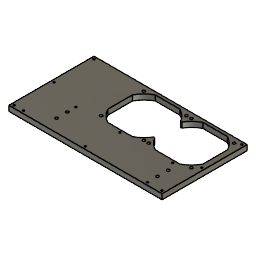
back (Autodesk Fusion 360 design; units mm, degrees)
Autodesk Fusion 360 part; units mm, degrees
sketch "Skizze1" plane through (0, 0, 0) normal (0, 0, 1) x (1, 0, 0)
  line L0 (258, 143.5) -> (0, 143.5)
  circle A0 centre (229, 39.5) radius 2.25
  circle A1 centre (229, 21.5) radius 2.25
  circle A2 centre (59, 54) radius 1.5
  circle A3 centre (4.5, 4.5) radius 1.5
  circle A4 centre (222, 54) radius 1.5
  circle A5 centre (4.5, 139) radius 1.5
  circle A6 centre (253.5, 4.5) radius 1.5
  circle A7 centre (253.5, 139) radius 1.5
  circle A8 centre (124.5, 4.5) radius 1.5
  circle A9 centre (253.5, 71.75) radius 1.5
  line L1 (0, 143.5) -> (0, 0)
  circle A10 centre (59, 39.5) radius 2.25
  circle A11 centre (20, 4.5) radius 1.5
  circle A12 centre (229, 4.5) radius 1.5
  circle A13 centre (59, 21.5) radius 2.25
  circle A14 centre (4.5, 71.75) radius 1.5
  line L2 (0, 143.5) -> (0, 0) construction
  line L3 (9, 143.5) -> (0, 143.5) construction
  circle A15 centre (133, 54) radius 1.5
  line L4 (0, 0) -> (258, 0)
  line L5 (0, 0) -> (9, 0) construction
  line L6 (258, 0) -> (258, 143.5)
  circle A16 centre (173.1, 134.4) radius 2.25
  arc A17 (210.3507, 143.5) -> (207.6493, 143.5) centre (209, 98.5) ccw construction
  arc A18 (249, 119.1597) -> (229.6597, 138.5) centre (209, 98.5) ccw
  arc A19 (188.3403, 138.5) -> (170.2508, 121.4199) centre (209, 98.5) ccw
  arc A20 (170.2508, 75.5801) -> (188.3403, 58.5) centre (209, 98.5) ccw
  arc A21 (229.6597, 58.5) -> (249, 77.8403) centre (209, 98.5) ccw
  circle A22 centre (244.9, 134.4) radius 2.25
  circle A23 centre (173.1, 62.6) radius 2.25
  circle A24 centre (244.9, 62.6) radius 2.25
  line L7 (188.3403, 138.5) -> (229.6597, 138.5)
  line L8 (249, 119.1597) -> (249, 77.8403)
  line L9 (188.3403, 58.5) -> (229.6597, 58.5)
  arc A25 (149.6597, 58.5) -> (167.7492, 75.5801) centre (129, 98.5) ccw
  arc A26 (167.7492, 121.4199) -> (149.6597, 138.5) centre (129, 98.5) ccw
  line L10 (108.3403, 138.5) -> (149.6597, 138.5)
  arc A27 (108.3403, 138.5) -> (89, 119.1597) centre (129, 98.5) ccw
  line L11 (89, 119.1597) -> (89, 77.8403)
  arc A28 (89, 77.8403) -> (108.3403, 58.5) centre (129, 98.5) ccw
  line L12 (108.3403, 58.5) -> (149.6597, 58.5)
  circle A29 centre (93.1, 134.4) radius 2.25
  circle A30 centre (93.1, 62.6) radius 2.25
  circle A31 centre (164.9, 62.6) radius 2.25
  circle A32 centre (164.9, 134.4) radius 2.25
  arc A33 (167.7492, 121.4199) -> (170.2508, 121.4199) centre (169, 122.1597) ccw
  arc A34 (170.2508, 75.5801) -> (167.7492, 75.5801) centre (169, 74.8403) ccw
  point P0 (253.5, 71.75)
  point P1 (253.5, 139)
  point P2 (253.5, 4.5)
  point P3 (253.5, 4.5)
  point P4 (253.5, 139)
  point P5 (253.5, 71.75)
  dimension "d1" = 143.5
  dimension "d2" = 258
  dimension "d6" = 18
  dimension "d7" = 4.5
  dimension "d8" = 4.5
  dimension "d9" = 4.5
  dimension "d10" = 4.5
  dimension "d11" = 3
  dimension "d12" = 3
  dimension "d13" = 3
  dimension "d14" = 3
  dimension "d15" = 3
  dimension "d22" = 20
  dimension "d24" = 209
  dimension "d26" = 104.5
  dimension "d27" = 3
  dimension "d28" = 3
  dimension "d29" = 3
  dimension "d30" = 67.25
  dimension "d31" = 9
  dimension "d32" = 67.25
  dimension "d33" = 67.25
  dimension "d34" = 3
  dimension "d35" = 3
  dimension "d36" = 3
  dimension "d37" = 67.25
  dimension "d45" = 2.25
  dimension "d47" = 4.5
  dimension "d48" = 4.5
  dimension "d49" = 4.5
  dimension "d50" = 2.25
  dimension "d51" = 4.5
  dimension "d52" = 4.5
  dimension "d53" = 4.5
  constraint horizontal L4
  constraint vertical L6
  constraint horizontal L0
  constraint vertical L1
  constraint coincident L1.end L2.end
  constraint horizontal L5
  constraint horizontal L3
  constraint vertical L2
  constraint coincident L0 A17.end
  constraint coincident L0 A17.start
  constraint concentric A17 A19
  constraint concentric A18 A19
  constraint concentric A19 A20
  constraint concentric A20 A21
  constraint concentric A26 A27
  constraint concentric A27 A28
  constraint concentric A25 A28
  constraint vertical L11
  constraint perpendicular L10 L11
  constraint tangent A19 A33
  measures "d1" distance of L0.end L1.end
  measures "d2" distance of L4.end L1.end
  measures "d6" distance of A13.centre A10.centre
  measures "d7" diameter of A10
  measures "d8" diameter of A13
  measures "d9" diameter of A0
  measures "d10" diameter of A1
  measures "d11" diameter of A15
  measures "d12" diameter of A2
  measures "d13" diameter of A4
  measures "d14" diameter of A11
  measures "d15" diameter of A8
  measures "d22" distance of A11.centre L1
  measures "d24" distance of A12.centre A11.centre
  measures "d26" distance of A8.centre A11.centre
  measures "d27" diameter of A6
  measures "d28" diameter of A7
  measures "d29" diameter of A9
  measures "d30" distance of P5 P1
  measures "d31" distance of L1.end L5.end
  measures "d32" distance of P4 P5
  measures "d33" distance of P5 P4
  measures "d34" diameter of A3
  measures "d35" diameter of A5
  measures "d36" diameter of A14
  measures "d37" distance of A5.centre A14.centre
  measures "d45" radius of A16
  measures "d47" diameter of A22
  measures "d48" diameter of A23
  measures "d49" diameter of A24
  measures "d50" radius of A29
  measures "d51" diameter of A32
  measures "d52" diameter of A30
  measures "d53" diameter of A31
extrude "Extrusion1" add sketch "Skizze1" along normal blind 9
